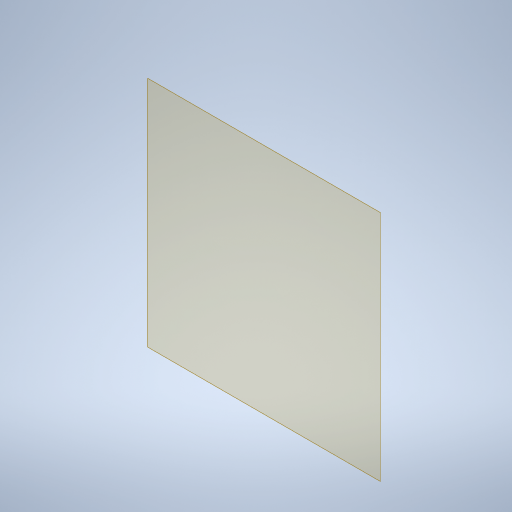
# Autodesk Inventor part: axle_cap
Saved by Autodesk Inventor 2024 (Build 280153000, 153)
## iProperties
Created: 2024-04-01
Part Number: axle_cap
Material: Generic
Document SubType Name: Modeling
Designer: MaartenGeorgesBuelen
Density: 1 g/cm^3
Appearance: Default
Author: MaartenGeorgesBuelen
## iProperties of the stored document axle_cap_3DPrint.ipt
Created: 2024-04-01
Part Number: axle_cap_3DPrint
Material: Generic
Document SubType Name: Modeling
Designer: MaartenGeorgesBuelen
Density: 1 g/cm^3
Appearance: Default
Author: MaartenGeorgesBuelen
Autodesk Inventor part; units mm, degrees
ref_plane "YZ Plane" through (0, 0, 0) normal (1, 0, 0) x (0, 1, 0)
ref_plane "XZ Plane" through (0, 0, 0) normal (0, 1, 0) x (-1, 0, 0)
ref_plane "XY Plane" through (0, 0, 0) normal (0, 0, 1) x (1, 0, 0)
ref_plane "Work Plane1" through (0, 0, -8) normal (0, 0, 1) x (1, 0, 0)
sketch "Sketch1" plane through (0, 0, -8) normal (0, 0, 1) x (1, 0, 0)
  circle A0 centre (0, 0) radius 13.09 projected
  circle A1 centre (0, 0) radius 10 projected
  circle A2 centre (0, 0) radius 13.09 projected
  circle A3 centre (0, 0) radius 10.3
  circle A4 centre (0, 0) radius 14.3
  line L0 (-7.8163, 11.9748) -> (-4.2157, 15.9521) construction
  line L1 (-4.2157, 15.9521) -> (-9.9494, 19.4831) construction
  spline S0 degree 2 poles (-7.8163, 11.9748) (-4.2157, 15.9521) (-9.9494, 19.4831) knots 1 1 1 2 2 2
  line L2 (-9.9494, 19.4831) -> (-9.2931, 20.5487)
  line L3 (-9.3147, 20.5137) -> (-3.3697, 16.8527) construction
  line L4 (-3.3697, 16.8527) -> (-4.8153, 13.4649) construction
  spline S1 degree 2 poles (-9.3147, 20.5137) (-3.3697, 16.8527) (-4.8153, 13.4649) knots 1 1 1 2 2 2
  line L5 (-4.8153, 13.4649) -> (-7.5493, 7.007)
  line L6 (0, 0) -> (0, 1.6434)
  line L7 (7.8163, 11.9748) -> (4.2157, 15.9521) construction
  line L8 (4.2157, 15.9521) -> (9.9494, 19.4831) construction
  spline S2 degree 2 poles (7.8163, 11.9748) (4.2157, 15.9521) (9.9494, 19.4831) knots 1 1 1 2 2 2
  line L9 (9.9494, 19.4831) -> (9.2931, 20.5487)
  line L10 (9.3147, 20.5137) -> (3.3697, 16.8527) construction
  line L11 (3.3697, 16.8527) -> (4.8153, 13.4649) construction
  spline S3 degree 2 poles (9.3147, 20.5137) (3.3697, 16.8527) (4.8153, 13.4649) knots 1 1 1 2 2 2
  line L12 (4.8153, 13.4649) -> (7.5493, 7.007)
  point P0 (0, 0)
  point P1 (4.8153, 13.4649)
  point P2 (7.5493, 7.007)
  point P3 (-4.8153, 13.4649)
  point P4 (7.8163, 11.9748)
  point P5 (4.8153, 13.4649)
  dimension "d0" = 0.3
  dimension "d1" = 4
  constraints: 10 end point, 9 symmetric about line, 2 point on circle, 2 point on line, 1 centre point, 1 perpendicular, 1 vertical, 15 other
extrude "Extrusion1" add sketch "Sketch1" along normal blind 2 contours A0 L5 A3 L12 | A0 L12 A4 L5 | S3 L9 S2 A4 | A4 S0 L2 S1 picked at (-7.0541, 9.7176) picked at (13.6381, 2.1556)
body "Solid1"
